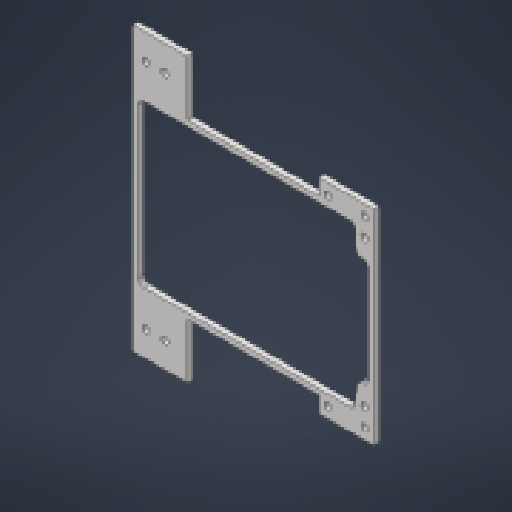
# Autodesk Inventor part: CeilUphold
Saved by Autodesk Inventor 2027.1 (Build 311270010, 270A)
## iProperties
Created: 2026-08-03
Part Number: CeilUphold
Material: Generic
Document SubType Name: Modeling
Designer: szymo
Density: 1 g/cm^3
Appearance: Default
Author: szymo
Autodesk Inventor part; units mm, degrees
ref_plane "YZ Plane" through (0, 0, 0) normal (1, 0, 0) x (0, 1, 0)
ref_plane "XZ Plane" through (0, 0, 0) normal (0, 1, 0) x (-1, 0, 0)
ref_plane "XY Plane" through (0, 0, 0) normal (0, 0, 1) x (1, 0, 0)
sketch "Sketch1" plane through (0, 0, 0) normal (0, 0, 1) x (1, 0, 0)
  circle A0 centre (3.25, 6.65) radius 1.2295 projected
  line L0 (0, 0) -> (6.5, 0) projected
  line L1 (6.5, 0) -> (6.5, 9.3) projected
  line L2 (6.5, 9.3) -> (0, 9.3) projected
  line L3 (0, 0) -> (0, 9.3) projected
  circle A1 centre (3.25, 13.15) radius 1.2295 projected
  line L4 (0, 9.3) -> (6.5, 9.3) projected
  line L5 (6.5, 9.3) -> (6.5, 17) projected
  line L6 (0, 17) -> (6.5, 17) projected
  line L7 (0, 9.3) -> (0, 17) projected
  circle A2 centre (3.25, -45.05) radius 1.2295 projected
  line L8 (0.5983, -42.4) -> (0, -42.4) projected
  line L9 (0, -42.4) -> (0, -47.7) projected
  line L10 (0, -47.7) -> (6.5, -47.7) projected
  line L11 (6.5, -38.4) -> (6.5, -47.7) projected
  line L12 (0.5983, -38.4) -> (6.5, -38.4) projected
  line L13 (0.5983, -38.4) -> (0.5983, -42.4) projected
  circle A3 centre (3.25, -51.55) radius 1.2295 projected
  line L14 (0, -47.7) -> (6.5, -47.7) projected
  line L15 (0, -47.7) -> (0, -55.4) projected
  line L16 (6.5, -55.4) -> (0, -55.4) projected
  line L17 (6.5, -47.7) -> (6.5, -55.4) projected
  circle A4 centre (-9.75, -51.55) radius 1.2295 projected
  line L18 (-41.3371, -47.7) -> (-6.5, -47.7) projected
  line L19 (-41.3371, -47.7) -> (-41.3371, -49.7) projected
  line L20 (-13, -49.7) -> (-41.3371, -49.7) projected
  line L21 (-13, -49.7) -> (-13, -55.4) projected
  line L22 (-6.5, -55.4) -> (-13, -55.4) projected
  line L23 (-6.5, -47.7) -> (-6.5, -55.4) projected
  circle A5 centre (-9.75, 13.15) radius 1.2295 projected
  line L24 (-41.3371, 11.3) -> (-13, 11.3) projected
  line L25 (-41.3371, 9.3) -> (-41.3371, 11.3) projected
  line L26 (-41.3371, 9.3) -> (-6.5, 9.3) projected
  line L27 (-6.5, 9.3) -> (-6.5, 17) projected
  line L28 (-13, 17) -> (-6.5, 17) projected
  line L29 (-13, 11.3) -> (-13, 17) projected
  arc A6 (-64.7971, 16.2257) -> (-64.1621, 16.7072) centre (-64.6621, 16.7072) ccw projected
  line L30 (-64.1621, 16.7072) -> (-64.1621, 23.8) projected
  arc A7 (-64.1621, 23.8) -> (-67.1621, 26.8) centre (-67.1621, 23.8) ccw projected
  line L31 (-67.1621, 26.8) -> (-70.1621, 26.8) projected
  line L32 (-70.1621, 26.8) -> (-70.1621, 29.3) projected
  line L33 (-70.1621, 29.3) -> (-59.3371, 29.3) projected
  line L34 (-59.3371, 29.3) -> (-59.3371, 30.8) projected
  line L35 (-59.3371, 30.8) -> (-78.8451, 30.8) projected
  line L36 (-78.8451, 16.3) -> (-78.8451, 30.8) projected
  line L37 (-65.3371, 16.3) -> (-78.8451, 16.3) projected
  arc A8 (-64.7971, 16.2257) -> (-65.3371, 16.3) centre (-65.3371, 14.3) ccw projected
  circle A9 centre (-67.4121, 21.8) radius 1.2295 projected
  circle A10 centre (-74.1621, 21.8) radius 1.2295 projected
  circle A11 centre (-67.4121, -60.2) radius 1.2295 projected
  circle A12 centre (-74.1621, -60.2) radius 1.2295 projected
  arc A13 (-64.1621, -55.1072) -> (-64.7971, -54.6257) centre (-64.6621, -55.1072) ccw projected
  arc A14 (-65.3371, -54.7) -> (-64.7971, -54.6257) centre (-65.3371, -52.7) ccw projected
  line L38 (-65.3371, -54.7) -> (-78.8451, -54.7) projected
  line L39 (-78.8451, -54.7) -> (-78.8451, -69.2) projected
  line L40 (-59.3371, -69.2) -> (-78.8451, -69.2) projected
  line L41 (-59.3371, -67.7) -> (-59.3371, -69.2) projected
  line L42 (-59.3371, -67.7) -> (-70.1621, -67.7) projected
  line L43 (-70.1621, -67.7) -> (-70.1621, -65.2) projected
  line L44 (-70.1621, -65.2) -> (-67.1621, -65.2) projected
  arc A15 (-67.1621, -65.2) -> (-64.1621, -62.2) centre (-67.1621, -62.2) ccw projected
  line L45 (-64.1621, -62.2) -> (-64.1621, -55.1072) projected
  line L46 (-59.3371, 30.8) -> (-59.3371, 11.3)
  line L47 (-59.3371, 11.3) -> (-41.3371, 11.3)
  line L48 (-41.3371, 9.3) -> (-76.8451, 9.3)
  line L49 (-78.8451, 16.3) -> (-78.8451, -54.7)
  line L50 (-76.8451, 9.3) -> (-76.8451, -47.7)
  line L51 (-76.8451, -47.7) -> (-41.3371, -47.7)
  line L52 (-41.3371, -49.7) -> (-59.3371, -49.7)
  line L53 (-59.3371, -49.7) -> (-59.3371, -67.7)
  line L54 (-6.5, 17) -> (0, 17)
  line L55 (-6.5, 9.3) -> (0, 9.3)
  line L56 (-6.5, -47.7) -> (0, -47.7)
  line L57 (-6.5, -55.4) -> (0, -55.4)
  line L58 (6.5, 0) -> (6.5, -38.4)
  line L59 (4.5, -38.4) -> (4.5, 0)
  dimension "d0" = 2
  dimension "d1" = 2
  constraints: 28 end point, 5 parallel, 5 perpendicular, 3 vertical, 2 point on line, 1 collinear, 1 horizontal
  measures "d0" distance from line of L36 L48.end
  measures "d1" distance between parallel lines of L58 L59
extrude "Extrusion1" add sketch "Sketch1" along normal blind 2 contours L3 L2 L1 L0 | L0 L58 L12 L59 | L7 L6 L5 L2 | L55 L27 L54 L7 | L12 L11 L10 L9 L8 L13 | L26 L25 L24 L29 L28 L27 | L48 L50 L51 L19 L52 L53 L42 L43 L44 A15 L45 A13 A14 L38 L49 L37 A8 A6 L30 A7 L31 L32 L33 L46 L47 L25 | L17 L16 L15 L10 | L15 L57 L23 L56 | L23 L22 L21 L20 L19 L18 | L33 L32 L31 A7 L30 A6 A8 L37 L36 L35 L34 | L41 L40 L39 L38 A14 A13 L45 A15 L44 L43 L42
fillet "Fillet1" radius 2 10 edges at (-76.8451, 9.3, 1) (-76.8451, -47.7, 1) (0.5983, -42.4, 1) (0, -42.4, 1) (0.5983, -38.4, 1) (4.5, -38.4, 1) (0, -47.7, 1) (0, 9.3, 1) (0, 0, 1) (4.5, 0, 1)
body "Solid1"
